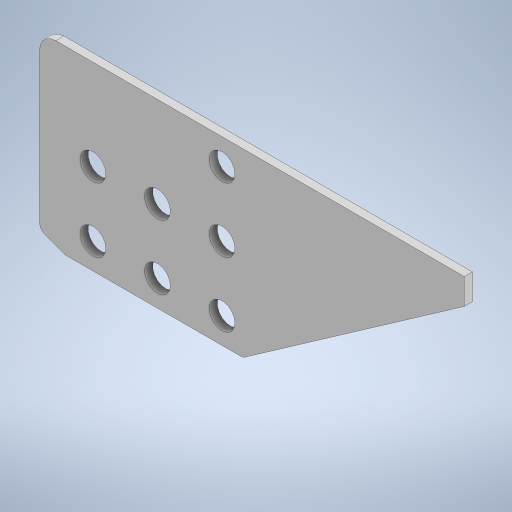
# Autodesk Inventor part: Sleds poly V3
Saved by Autodesk Inventor 2023 (Build 270158000, 158)
## iProperties
Created: 2024-01-28
Part Number: Sleds poly V3
Material: Generic
Document SubType Name: Modeling
Designer: diego
Density: 1 g/cm^3
Appearance: Default
Author: diego
Autodesk Inventor part; units mm, degrees
ref_plane "YZ Plane" through (0, 0, 0) normal (1, 0, 0) x (0, 1, 0)
ref_plane "XZ Plane" through (0, 0, 0) normal (0, 1, 0) x (-1, 0, 0)
ref_plane "XY Plane" through (0, 0, 0) normal (0, 0, 1) x (1, 0, 0)
sketch "Sketch1" plane through (0, 0, 0) normal (0, 0, 1) x (1, 0, 0)
  line L0 (0, 0) -> (-114.4136, 0)
  line L1 (0, 51.7869) -> (-1.5875, 51.7869)
  line L2 (-1.5875, 51.7869) -> (-4.1188, 51.7869)
  circle A0 centre (-4.1188, 51.7869) radius 2.54
  line L3 (-4.1188, 51.7869) -> (-16.8188, 51.7869)
  circle A1 centre (-16.8188, 51.7869) radius 2.54
  line L4 (-16.8188, 51.7869) -> (-29.5188, 51.7869)
  circle A2 centre (-29.5188, 51.7869) radius 2.54
  line L5 (-4.1188, 51.7869) -> (-4.1188, 39.0869)
  circle A3 centre (-4.1188, 39.0869) radius 2.54
  line L6 (-4.1188, 39.0869) -> (0, 39.0869)
  line L7 (-4.1188, 39.0869) -> (-4.1188, 34.0008)
  line L8 (-4.1188, 34.0008) -> (0, 34.0008)
  line L9 (0, 34.0008) -> (61.785, 77.2755)
  line L10 (-4.1188, 51.7869) -> (-4.1188, 64.4869)
  circle A4 centre (-4.1188, 64.4869) radius 2.54
  line L11 (-4.1188, 64.4869) -> (0, 64.4869)
  line L12 (0, 64.4869) -> (43.5263, 64.4869)
  line L13 (-29.5188, 51.7869) -> (-84.2272, 51.7869)
  line L14 (-29.5188, 51.7869) -> (-29.5188, 39.0869)
  line L15 (-16.8188, 51.7869) -> (-16.8188, 39.0869)
  circle A5 centre (-29.5188, 39.0869) radius 2.54
  circle A6 centre (-16.8188, 39.0869) radius 2.54
  line L16 (-4.1188, 34.0008) -> (-34.9438, 34.0008)
  line L17 (-34.9438, 34.0008) -> (-84.2272, 51.7869)
  line L18 (-4.1188, 64.4869) -> (-4.1188, 69.5669)
  line L19 (-4.1188, 64.4869) -> (-40.0106, 51.7869)
  line L20 (-40.0106, 51.7869) -> (-40.0106, 35.8294)
  line L21 (-4.1188, 69.5669) -> (50.7792, 69.5669)
  line L22 (43.5263, 64.4869) -> (43.5263, 69.5669)
  line L23 (-4.1188, 69.5669) -> (-40.0106, 69.5669)
  line L24 (-40.0106, 51.7869) -> (-40.0106, 69.5669)
  line L25 (-48.9201, 51.7869) -> (-4.1188, 69.5669)
  dimension "d22" = 1.5875
  dimension "d23" = 5.08
  dimension "d24" = 12.7
  dimension "d25" = 5.08
  dimension "d26" = 12.7
  dimension "d27" = 5.08
  dimension "d28" = 12.7
  dimension "d29" = 5.08
  dimension "d30" = 12.7
  dimension "d31" = 5.08
  dimension "d32" = 5.08
  dimension "d33" = 5.08
  dimension "d34" = 5.08
  constraints: 52 end point, 11 horizontal, 8 point on line, 7 centre point, 7 coincident, 7 vertical, 3 perpendicular
  measures "d22" distance of L1.start L1.end
  measures "d23" diameter of A0
  measures "d24" distance of L3.start L3.end
  measures "d25" diameter of A1
  measures "d26" distance of L4.start L4.end
  measures "d27" diameter of A2
  measures "d28" distance of L3.start L5.end
  measures "d29" diameter of A3
  measures "d30" distance of L3.start L10.end
  measures "d31" diameter of A4
  measures "d32" diameter of A5
  measures "d33" diameter of A6
  measures "d34" distance of L11.start L18.end
extrude "Extrusion2" add sketch "Sketch1" along normal blind 1.5875 contours A0 L10 A4 L11 L12 L9 L8 L7 A3 L5 | A0 L3 A1 L4 A2 L13 L19 A4 L10 | L5 A3 L7 L16 L17 L20 L13 A2 L4 A1 L3 A0 | L19 L24 L25 L18 A4 | A4 L18 L21 L22 L12 L11 | L25 L24 L23
fillet "Fillet7" radius 1.5875 3 edges at (0, 34.0008, 0.7937) (-40.0106, 35.8294, 0.7937) (-34.9438, 34.0008, 0.7937)
fillet "Fillet8" radius 3.175 1 edges at (-40.0106, 69.5669, 0.7937)
body "Solid2"
